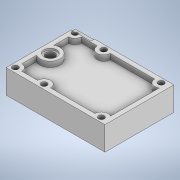
# Autodesk Inventor part: HousingVX
Saved by Autodesk Inventor 2020 (Build 240168000, 168)
## iProperties
Created: 2020-06-15
Part Number: HousingVX
Material: Generic
Document SubType Name: Modeling
Designer: Admin
Density: 1 g/cm^3
Appearance: Default
Author: Admin
Autodesk Inventor part; units mm, degrees
ref_plane "YZ Plane" through (0, 0, 0) normal (1, 0, 0) x (0, 1, 0)
ref_plane "XZ Plane" through (0, 0, 0) normal (0, 1, 0) x (-1, 0, 0)
ref_plane "XY Plane" through (0, 0, 0) normal (0, 0, 1) x (1, 0, 0)
sketch "Sketch1" plane through (0, 0, 0) normal (0, 1, 0) x (-1, 0, 0)
  line L0 (0, 0) -> (54.67, 0)
  line L1 (54.67, 0) -> (54.67, -38.1)
  line L2 (54.67, -38.1) -> (0, -38.1)
  line L3 (0, -38.1) -> (0, 0)
  dimension "d0" = 54.67
  dimension "d1" = 38.1
  constraints: 8 end point, 2 parallel, 1 horizontal, 1 perpendicular
  measures "d0" distance of L1.end L2.end
  measures "d1" distance of L2.end L0.start
extrude "Extrusion1" add sketch "Sketch1" along normal blind 13.2
sketch "Sketch2" plane through (0, 13.2, 0) normal (0, 1, 0) x (1, 0, 0)
  circle A0 centre (-52.13, 2.54) radius 1.6
  circle A1 centre (-36.25, 2.54) radius 1.6
  circle A2 centre (-4.5, 2.54) radius 1.6
  circle A3 centre (-52.13, 35.56) radius 1.6
  circle A4 centre (-36.25, 35.56) radius 1.6
  circle A5 centre (-4.5, 35.56) radius 1.6
  line L0 (-54.67, 0) -> (0, 0)
  line L1 (0, 38.1) -> (-54.67, 38.1)
  line L2 (-54.67, 38.1) -> (-54.67, 0)
  line L3 (0, 0) -> (0, 38.1)
  dimension "d4" = 3.2
  dimension "d5" = 3.2
  dimension "d6" = 3.2
  dimension "d7" = 3.2
  dimension "d8" = 3.2
  dimension "d9" = 3.2
  dimension "d10" = 2.54
  dimension "d11" = 2.54
  dimension "d12" = 2.54
  dimension "d13" = 2.54
  dimension "d14" = 2.54
  dimension "d15" = 2.54
  dimension "d16" = 2.54
  dimension "d17" = 4.5
  dimension "d18" = 36.25
  dimension "d19" = 4.5
  dimension "d20" = 36.25
  dimension "d21" = 2.54
  constraints: 8 end point, 6 centre point
  measures "d4" diameter of A0
  measures "d5" diameter of A1
  measures "d6" diameter of A2
  measures "d7" diameter of A3
  measures "d8" diameter of A4
  measures "d9" diameter of A5
  measures "d10" distance from line of L0 A0.centre
  measures "d11" distance from line of L0 A1.centre
  measures "d12" distance from line of L0 A2.centre
  measures "d13" distance from line of L1 A3.centre
  measures "d14" distance from line of L1 A4.centre
  measures "d15" distance from line of L1 A5.centre
  measures "d16" distance from line of L2 A0.centre
  measures "d17" distance from line of L3 A2.centre
  measures "d18" distance from line of L3 A1.centre
  measures "d19" distance from line of L3 A5.centre
  measures "d20" distance from line of L3 A4.centre
  measures "d21" distance from line of L2 A3.centre
extrude "Extrusion2" cut sketch "Sketch2" against normal through all contours A0 | A1 | A2 | A3 | A4 | A5
sketch "Sketch3" plane through (0, 13.2, 0) normal (0, 1, 0) x (1, 0, 0)
  arc A0 (-52.13, 31.96) -> (-48.53, 35.56) centre (-52.13, 35.56) ccw
  arc A1 (-39.85, 35.56) -> (-32.65, 35.56) centre (-36.25, 35.56) ccw
  arc A2 (-8.1, 35.56) -> (-2.54, 32.5403) centre (-4.5, 35.56) ccw
  arc A3 (-2.54, 5.5597) -> (-8.1, 2.54) centre (-4.5, 2.54) ccw
  arc A4 (-32.65, 2.54) -> (-39.85, 2.54) centre (-36.25, 2.54) ccw
  arc A5 (-48.53, 2.54) -> (-52.13, 6.14) centre (-52.13, 2.54) ccw
  arc A6 (-52.13, 14.2583) -> (-52.13, 23.8417) centre (-49.43, 19.05) ccw
  line L0 (-48.53, 35.56) -> (-39.85, 35.56)
  line L1 (-32.65, 35.56) -> (-8.1, 35.56)
  line L2 (-2.54, 32.5403) -> (-2.54, 5.5597)
  line L3 (-52.13, 14.2583) -> (-52.13, 6.14)
  line L4 (-48.53, 2.54) -> (-39.85, 2.54)
  line L5 (-32.65, 2.54) -> (-8.1, 2.54)
  line L6 (0, 0) -> (0, 38.1)
  line L7 (0, 38.1) -> (-54.67, 38.1)
  line L8 (-54.67, 0) -> (0, 0)
  line L9 (-54.67, 38.1) -> (-54.67, 0)
  line L10 (-52.13, 31.96) -> (-52.13, 23.8417)
  dimension "d24" = 4.5
  dimension "d25" = 2.54
  dimension "d26" = 2.54
  dimension "d27" = 4.5
  dimension "d28" = 2.54
  dimension "d29" = 36.25
  dimension "d30" = 15.88
  dimension "d31" = 36.25
  dimension "d32" = 15.88
  dimension "d33" = 2.54
  dimension "d34" = 2.54
  dimension "d35" = 2.54
  dimension "d36" = 3.6
  dimension "d37" = 3.6
  dimension "d38" = 3.6
  dimension "d39" = 3.6
  dimension "d40" = 3.6
  dimension "d41" = 3.6
  dimension "d42" = 2.54
  dimension "d43" = 2.54
  dimension "d44" = 2.54
  dimension "d45" = 2.54
  dimension "d46" = 2.54
  dimension "d47" = 2.54
  dimension "d48" = 2.54
  dimension "d49" = 5.24
  dimension "d50" = 19.05
  dimension "d51" = 5.5
  constraints: 22 end point, 14 point on circle, 7 centre point, 4 horizontal, 3 vertical
  measures "d24" distance from line of L6 A2.centre
  measures "d25" distance from line of L7 A2.centre
  measures "d26" distance from line of L8 A3.centre
  measures "d27" distance from line of L6 A3.centre
  measures "d28" distance from line of L8 A4.centre
  measures "d29" distance from line of L6 A4.centre
  measures "d30" distance of A4.centre A5.centre
  measures "d31" distance from line of L6 A1.centre
  measures "d32" distance of A1.centre A0.centre
  measures "d33" distance from line of L7 A0.centre
  measures "d34" distance from line of L7 A1.centre
  measures "d35" distance from line of L8 A5.centre
  measures "d36" radius of A0
  measures "d37" radius of A1
  measures "d38" radius of A2
  measures "d39" radius of A3
  measures "d40" radius of A4
  measures "d41" radius of A5
  measures "d42" distance between parallel lines of L7 L0
  measures "d43" distance between parallel lines of L7 L1
  measures "d44" distance between parallel lines of L8 L4
  measures "d45" distance between parallel lines of L6 L2
  measures "d46" distance between parallel lines of L8 L5
  measures "d47" distance between parallel lines of L9 L3
  measures "d48" distance between parallel lines of L9 L10
  measures "d49" distance from line of L9 A6.centre
  measures "d50" distance from line of L8 A6.centre
  measures "d51" radius of A6
extrude "Extrusion3" cut sketch "Sketch3" against normal blind 3 contours A0 L0 A1 L1 A2 L2 A3 L5 A4 L4 A5 L3 A6 L10
sketch "Sketch5" plane through (0, 13.2, 0) normal (0, 1, 0) x (1, 0, 0)
  circle A0 centre (-49.27, 19.05) radius 3.5
  line L0 (-54.67, 38.1) -> (-54.67, 0) projected
  line L1 (-54.67, 0) -> (0, 0) projected
  dimension "d61" = 7
  dimension "d62" = 5.4
  dimension "d63" = 19.05
  constraints: 1 centre point
  measures "d61" diameter of A0
  measures "d62" distance from line of L0 A0.centre
  measures "d63" distance from line of A0.centre L1
extrude "Extrusion5" cut sketch "Sketch5" against normal blind 0.9
sketch "Sketch15" plane through (-49.27, 12.3, -19.05) normal (0, 1, 0) x (1, 0, 0)
  circle A0 centre (0, 0) radius 2.5
  line L0 (-5.4, 19.05) -> (-5.4, -19.05) projected
  line L1 (49.27, 19.05) -> (-5.4, 19.05) projected
  point P0 (49.27, -19.05)
  dimension "d116" = 5
  dimension "d117" = 5.4
  dimension "d118" = 19.05
  constraints: 1 centre point
  measures "d116" diameter of A0
  measures "d117" distance from line of L0 A0.centre
  measures "d118" distance from line of L1 A0.centre
extrude "Extrusion13" cut sketch "Sketch15" against normal through all
sketch "Sketch18" plane through (0, 0, -38.1) normal (0, 0, -1) x (-1, 0, 0)
  circle A0 centre (49.27, 8.2) radius 1
  line L0 (54.67, 0) -> (54.67, 13.2) projected
  line L1 (0, 13.2) -> (54.67, 13.2) projected
  point P0 (0, 0)
  dimension "d124" = 2
  dimension "d125" = 5.4
  dimension "d126" = 5
  constraints: 1 centre point
  measures "d124" diameter of A0
  measures "d125" distance from line of L0 A0.centre
  measures "d126" distance from line of A0.centre L1
extrude "Extrusion14" cut sketch "Sketch18" against normal blind 19
sketch "Sketch20" plane through (-54.67, 0, -38.1) normal (-1, 0, 0) x (0, 0, 1)
  line L0 (2, 13.2) -> (0, 13.2)
  line L1 (0, 13.2) -> (0, 12.7)
  line L2 (0, 12.7) -> (2, 12.2)
  line L3 (2, 12.2) -> (2, 13.2)
  point P0 (38.1, 0)
  dimension "d129" = 0.5
  dimension "d130" = 1
  dimension "d131" = 2
  constraints: 8 end point, 1 coincident, 1 horizontal, 1 parallel, 1 perpendicular
  measures "d129" distance of L0.end L1.end
  measures "d130" distance of L2.end L0.start
  measures "d131" distance of L0.start L0.end
extrude "Extrusion15" cut sketch "Sketch20" against normal blind 10.8
sketch "Sketch21" plane through (0, 0, -38.1) normal (0, 0, -1) x (-1, 0, 0)
  circle A0 centre (49.27, 8.2) radius 3.5
  line L0 (54.67, 0) -> (54.67, 12.7) projected
  line L1 (43.87, 13.2) -> (50.6239, 13.2) projected
  point P0 (0, 0)
  dimension "d134" = 7
  dimension "d135" = 5.4
  dimension "d136" = 5
  constraints: 1 centre point
  measures "d134" diameter of A0
  measures "d135" distance from line of L0 A0.centre
  measures "d136" distance from line of A0.centre L1
extrude "Extrusion16" cut sketch "Sketch21" against normal blind 0.9
body "Solid1"
